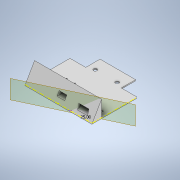
# Autodesk Inventor part: Onixium3
Saved by Autodesk Inventor 2021 (Build 250183000, 183)
## iProperties
Created: 2021-11-17
Part Number: Onixium3
Material: Genérico
Document SubType Name: Chapa
Designer: Juan Camilo
Density: 1 g/cm^3
Sheet Metal Rule: Por defecto_mm
Appearance: Valor por defecto
Author: Juan Camilo
Autodesk Inventor part; units mm, degrees
ref_plane "YZ Plane" through (0, 0, 0) normal (1, 0, 0) x (0, 1, 0)
ref_plane "XZ Plane" through (0, 0, 0) normal (0, 1, 0) x (-1, 0, 0)
ref_plane "XY Plane" through (0, 0, 0) normal (0, 0, 1) x (1, 0, 0)
sketch "Boceto1" plane through (0, 0, 0) normal (0, 1, 0) x (-1, 0, 0)
  line L0 (26, -66) -> (49, -66)
  line L1 (0, -87) -> (0, 0) construction
  line L2 (49, 0) -> (49, -87)
  line L3 (-49, 0) -> (49, 0)
  line L4 (-49, -87) -> (-49, 0)
  line L5 (49, -87) -> (-49, -87)
  line L6 (26, -87) -> (26, -66)
  circle A0 centre (-41.5, -7.5) radius 1.75
  line L7 (49, -12) -> (-49, -12) construction
  circle A1 centre (41.5, -7.5) radius 1.75
  line L8 (-26, -66) -> (-49, -66)
  line L9 (-26, -87) -> (-26, -66)
  line L10 (44.5, -24.05) -> (28.5, -24.05)
  line L11 (28.5, -24.05) -> (28.5, -13.05)
  line L12 (28.5, -13.05) -> (44.5, -13.05)
  line L13 (44.5, -13.05) -> (44.5, -24.05)
  line L14 (42.5, -23.55) -> (31.5, -23.55)
  line L15 (31.5, -14.85) -> (42.5, -14.85)
  line L16 (42.5, -14.85) -> (42.5, -23.55)
  circle A2 centre (30.2, -19.25) radius 1.05
  line L17 (31.5, -14.85) -> (31.5, -23.55)
  line L18 (-42.5, -23.55) -> (-31.5, -23.55)
  line L19 (-42.5, -14.85) -> (-42.5, -23.55)
  line L20 (-31.5, -14.85) -> (-42.5, -14.85)
  line L21 (-31.5, -14.85) -> (-31.5, -23.55)
  circle A3 centre (-30.2, -19.25) radius 1.05
  circle A4 centre (13, -21.5) radius 2.5
  circle A5 centre (-13, -21.5) radius 2.5
  circle A6 centre (16, -70) radius 2.5
  circle A7 centre (-16, -70) radius 2.5
  dimension "d0" = 3.5
  dimension "d1" = 0
  dimension "d2" = 87
  dimension "d3" = 21
  dimension "d4" = 12
  dimension "d5" = 23
  dimension "d6" = 98
  dimension "d7" = 7.5
  dimension "d8" = 7.5
  dimension "d9" = 79.5
  dimension "d10" = 2.1
  dimension "d11" = 9
  dimension "d12" = 11
  dimension "d13" = 16
  dimension "d14" = 1
  dimension "d15" = 3.6
  dimension "d16" = 2.1
  dimension "d17" = 1.3
  dimension "d18" = 5
  dimension "d19" = 36
  dimension "d20" = 9.5
  dimension "d21" = 5
  dimension "d22" = 17
  dimension "d23" = 10
  dimension "d24" = 8.7
  dimension "d25" = 4.3
  dimension "d26" = 4
  dimension "d27" = 11
  dimension "d28" = 54
  dimension "d29" = 2.85
  constraints: 44 end point, 10 symmetric about line, 8 centre point, 5 parallel, 5 point on line, 4 horizontal, 4 perpendicular, 3 midpoint, 1 equal radius, 1 vertical, 3 other
  measures "d0" diameter of A0
  measures "d1" distance of point (0, 0) L1.end
  measures "d2" distance of L2.start L2.end
  measures "d3" distance of L6.start L0.start
  measures "d4" distance between parallel lines of L3 L7
  measures "d5" distance of L0.start L0.end
  measures "d6" distance of L4.end L2.start
  measures "d7" distance from line of L2 A1.centre
  measures "d8" distance from line of L3 A1.centre
  measures "d10" diameter of L7 L12
  measures "d11" diameter of L2 L13
  measures "d12" distance of L11.start L11.end
  measures "d13" distance of L10.start L11.start
  measures "d14" diameter of L14 L10
  measures "d15" diameter of L15 L12
  measures "d16" diameter of A2
  measures "d17" distance from line of L17 A2.centre
  measures "d18" diameter of A4
  measures "d19" distance from line of L2 A4.centre
  measures "d20" distance from line of L7 A4.centre
  measures "d21" diameter of A6
  measures "d22" distance from line of L5 A6.centre
  measures "d23" distance from line of L6 A6.centre
  measures "d24" distance of L17.start L17.end
  measures "d25" distance from line of L14 A2.centre
  measures "d26" diameter of L16 L13
  measures "d27" distance of L17.start L15.end
  measures "d28" distance between parallel lines of L7 L0
  measures "d29" distance between parallel lines of L7 L15
extrude "Base" add sketch "Boceto1" along normal blind 1.5 contours L6 L5 L9 L8 L4 L3 L2 L0 | L10 L11 L12 L13
sketch "Boceto2" plane through (-49, 0, -66) normal (-1, 0, 0) x (0, 0, 1)
  line L0 (66, 0) -> (0, 0)
  line L1 (66, 0) -> (65.1357, 1.5)
  line L2 (66, 0) -> (67.7312, 0) construction
  line L3 (65.1357, 1.5) -> (66, 1.5)
  line L4 (66, 0) -> (66, 1.5)
  line L5 (66, 1.5) -> (66, 0)
  dimension "d32" = 119.95
  constraints: 12 end point, 2 horizontal, 1 equal length, 1 perpendicular
  measures "d32" angle of L2 L1
extrude "Angulo Base" cut sketch "Boceto2" against normal blind 98
sketch "Boceto3" plane through (-49, 0, -66) normal (-1, 0, 0) x (0, 0, 1)
  line L0 (0, 0) -> (66, 0) projected
  line L1 (51.8028, 0) -> (66, 0)
  line L2 (66, 0) -> (51.8028, 24.6399)
  line L3 (51.8028, 24.6399) -> (51.8028, 0)
  line L4 (66, 0) -> (65.1357, 1.5) projected
  dimension "d35" = 0
  constraints: 6 end point, 1 collinear, 1 perpendicular, 1 point on line
  measures "d35" distance between parallel lines of L4 L2
extrude "Extrusión3" add sketch "Boceto3" against normal blind 98
sketch "Boceto4" plane through (-49, 1.5, -14.1972) normal (0, 0, -1) x (-1, 0, 0)
  line L0 (-55.5, 19.6399) -> (-42.5, 19.6399)
  line L1 (-42.5, 19.6399) -> (-42.5, 0.9399)
  line L2 (-42.5, 0.9399) -> (-55.5, 0.9399)
  line L3 (-55.5, 0.9399) -> (-55.5, 19.6399)
  line L4 (-54.6, 10.4399) -> (-43.4, 10.4399)
  line L5 (-43.4, 10.4399) -> (-43.4, 4.8399)
  line L6 (-43.4, 4.8399) -> (-54.6, 4.8399)
  line L7 (-54.6, 4.8399) -> (-54.6, 10.4399)
  line L8 (0, 23.1399) -> (0, 0) projected
  line L9 (-98, 0) -> (-98, 23.1399) projected
  line L10 (0, 23.1399) -> (-98, 23.1399) projected
  line L11 (0, 0) -> (-98, 0) projected
  point P0 (-49, -1.5)
  dimension "d38" = 13
  dimension "d39" = 0.9
  dimension "d40" = 0.9
  dimension "d41" = 3.9
  dimension "d42" = 5.6
  dimension "d43" = 18.7
  dimension "d44" = 42.5
  dimension "d45" = 42.5
  dimension "d46" = 3.5
  dimension "d93" = 0.9399
  constraints: 16 end point, 4 parallel, 2 horizontal, 2 perpendicular
  measures "d38" distance between parallel lines of L1 L3
  measures "d39" distance between parallel lines of L3 L7
  measures "d40" distance between parallel lines of L1 L5
  measures "d41" distance between parallel lines of L2 L6
  measures "d42" distance between parallel lines of L6 L4
  measures "d43" distance between parallel lines of L2 L0
  measures "d44" distance between parallel lines of L8 L1
  measures "d45" distance between parallel lines of L9 L3
  measures "d46" distance between parallel lines of L0 L10
  measures "d93" distance between parallel lines of L11 L2
extrude "Extrusión4" cut sketch "Boceto4" against normal mid plane 76.25 contours L4 L5 L6 L7
sketch "Boceto5" plane through (-49, 1.5, -14.1972) normal (0, 0, -1) x (-1, 0, 0)
  line L0 (-54.6, 19.64) -> (-43.4, 19.64)
  line L1 (-43.4, 19.64) -> (-43.4, 4.84)
  line L2 (-43.4, 4.84) -> (-54.6, 4.84)
  line L3 (-54.6, 4.84) -> (-54.6, 19.64)
  line L4 (-54.6, 4.8399) -> (-54.6, 10.4399) projected
  line L5 (-43.4, 10.4399) -> (-43.4, 4.8399) projected
  line L6 (-43.4, 4.8399) -> (-54.6, 4.8399) projected
  line L7 (-75, 0) -> (-23, 0) projected
  line L8 (0, 23.1399) -> (-98, 23.1399) projected
  point P0 (-49, -1.5)
  dimension "d49" = 11.2
  dimension "d50" = 14.8
  dimension "d76" = 4.84
  constraints: 8 end point, 2 parallel, 1 horizontal, 1 perpendicular
  measures "d49" distance between parallel lines of L1 L3
  measures "d50" distance between parallel lines of L2 L0
  measures "d76" distance between parallel lines of L7 L2
extrude "Extrusión5" cut sketch "Boceto5" against normal mid plane 1.5
sketch "Boceto6" plane through (0, 1.5, 0) normal (0, 1, 0) x (1, 0, 0)
  line L0 (6.5, 13.7984) -> (-6.5, 13.7984)
  line L1 (-6.5, 13.7984) -> (-6.5, 13.8318)
  line L2 (-6.5, 13.8318) -> (6.5, 13.8318)
  line L3 (6.5, 13.8318) -> (6.5, 13.7984)
  line L4 (-6.5, 13.8318) -> (6.5, 13.8318)
  line L5 (6.5, 13.8318) -> (6.5, 18.6972)
  line L6 (6.5, 18.6972) -> (-6.5, 18.6972)
  line L7 (-6.5, 18.6972) -> (-6.5, 13.8318)
  line L8 (-49, 14.1972) -> (49, 14.1972) projected
  point P0 (0, 0)
  point P1 (-6.5, 14.1972)
  point P2 (6.5, 14.1972)
  dimension "d53" = 13
  dimension "d54" = 4.5
  constraints: 16 end point, 4 parallel, 2 horizontal, 2 perpendicular, 1 point on line
  measures "d53" distance between parallel lines of L7 L5
  measures "d54" distance between parallel lines of L8 L6
extrude "Extrusión6" add sketch "Boceto6" along normal blind 20 contours L8 L7 L6 L5
sketch "Boceto7" plane through (6.5, 1.5, -18.6972) normal (0, 0, -1) x (-1, 0, 0)
  line L0 (0.9, 10.916) -> (12.1, 10.916)
  line L1 (12.1, 10.916) -> (12.1, 4.84)
  line L2 (12.1, 4.84) -> (0.9, 4.84)
  line L3 (0.9, 4.84) -> (0.9, 10.916)
  line L4 (13, 0) -> (0, 0) projected
  line L5 (0, 0) -> (0, 20) projected
  line L6 (0.9, 20) -> (12.1, 20)
  line L7 (12.1, 20) -> (12.1, 15.894)
  line L8 (12.1, 15.894) -> (0.9, 15.894)
  line L9 (0.9, 15.894) -> (0.9, 20)
  line L10 (0, 20) -> (13, 20) projected
  point P0 (6.5, -1.5)
  dimension "d57" = 4.84
  dimension "d58" = 6.076
  dimension "d59" = 11.2
  dimension "d60" = 0.9
  dimension "d61" = 4.978
  dimension "d62" = 11.2
  dimension "d63" = 0.9
  dimension "d64" = 0
  constraints: 16 end point, 4 parallel, 2 horizontal, 2 perpendicular
  measures "d57" distance between parallel lines of L4 L2
  measures "d58" distance between parallel lines of L2 L0
  measures "d59" distance between parallel lines of L1 L3
  measures "d60" distance between parallel lines of L5 L3
  measures "d61" distance between parallel lines of L8 L0
  measures "d62" distance between parallel lines of L7 L9
  measures "d63" distance between parallel lines of L5 L9
  measures "d64" distance between parallel lines of L10 L6
extrude "Extrusión7" cut sketch "Boceto7" against normal blind 5.25
sketch "Boceto8" plane through (-5.6, 17.394, -18.6972) normal (0, 1, 0) x (1, 0, 0)
  line L0 (0, 0) -> (0, -4.5) projected
  line L1 (0, -4.5) -> (11.2, -4.5)
  line L2 (11.2, -4.5) -> (11.2, -0.7)
  line L3 (11.2, -0.7) -> (0, -0.7)
  line L4 (0, -0.7) -> (0, -4.5)
  point P0 (5.6, -18.6972)
  point P1 (0, -0.7)
  dimension "d67" = 3.8
  dimension "d68" = 11.2
  constraints: 8 end point, 2 parallel, 1 horizontal, 1 perpendicular
  measures "d67" distance between parallel lines of L3 L1
  measures "d68" distance between parallel lines of L0 L2
extrude "Extrusión8" cut sketch "Boceto8" against normal blind 10.054
sketch "Boceto9" plane through (-5.6, 6.34, -18.6972) normal (0, 1, 0) x (1, 0, 0)
  line L0 (11.2, 0) -> (11.2, -0.7) projected
  line L1 (0, 0) -> (0, -4.5) projected
  line L2 (11.2, -0.7) -> (0, -0.7)
  line L3 (0, -0.7) -> (0, -1.7)
  line L4 (0, -1.7) -> (11.2, -1.7)
  line L5 (11.2, -1.7) -> (11.2, -0.7)
  point P0 (5.6, -18.6972)
  dimension "d77" = 1
  constraints: 8 end point, 2 parallel, 1 horizontal, 1 perpendicular, 1 point on line
  measures "d77" distance between parallel lines of L4 L2
extrude "Extrusión9" cut sketch "Boceto9" against normal blind 3.9
sketch "Boceto12" plane through (0, 1.5, 0) normal (0, 1, 0) x (1, 0, 0)
  line L0 (-49, 0) -> (49, 0) projected
  line L1 (16.0988, 0) -> (49, 15.3421)
  line L2 (49, 0) -> (49, 66) projected
  point P0 (0, 0)
  dimension "d82" = 25
  constraints: 2 end point, 2 point on line
  measures "d82" angle of L0 L1
ref_plane "Plano de trabajo1" through (16.0988, 1.5, 0) normal (-0.4226183, 0, -0.9063078) x (0.9063078, 0, -0.4226183)
sketch "Boceto13" plane through (16.0988, 1.5, 0) normal (-0.4226183, 0, -0.9063078) x (0.9063078, 0, -0.4226183)
  line L0 (20.8186, -18.14) -> (9.6186, -18.14)
  line L1 (9.6186, -18.14) -> (9.6186, 0.56)
  line L2 (9.6186, 0.56) -> (20.8186, 0.56)
  line L3 (20.8186, 0.56) -> (20.8186, -18.14)
  line L4 (22.8276, -9.416) -> (9.6186, -9.416)
  line L5 (9.6186, -9.416) -> (9.6186, -3.34)
  line L6 (9.6186, -3.34) -> (22.8276, -3.34)
  line L7 (22.8276, -3.34) -> (22.8276, -9.416)
  line L8 (35.8186, 0) -> (35.8186, -23.1399) projected
  line L9 (-58.9996, 1.5) -> (29.8186, 1.5) projected
  point P0 (-14.5905, 1.5)
  point P1 (9.6186, -9.416)
  dimension "d84" = 18.7
  dimension "d85" = 11.2
  dimension "d86" = 6.076
  dimension "d87" = 0
  dimension "d88" = 3.9
  dimension "d91" = 15
  dimension "d92" = 0.94
  constraints: 16 end point, 4 parallel, 2 horizontal, 2 perpendicular
  measures "d84" distance between parallel lines of L2 L0
  measures "d85" distance between parallel lines of L1 L3
  measures "d86" distance between parallel lines of L6 L4
  measures "d87" distance between parallel lines of L1 L5
  measures "d88" distance between parallel lines of L2 L6
  measures "d91" distance between parallel lines of L8 L3
  measures "d92" distance between parallel lines of L9 L2
extrude "Extrusión10" cut sketch "Boceto13" against normal mid plane 45.15 contours L4 L1 L6 L3 | L3 L6 L7 L4
equation "\"Radio_pliegue\" = Grosor"
equation "\"Anchura_desahogo_plegado\" = Grosor"
equation "\"Profundidad_desahogo_plegado\" = 0.5 * Grosor"
equation "\"Tamaño_destalonado\" = 4 * Grosor"
equation "\"Remanente_mínimo\" = 2 * Grosor"
equation "\"Radiodetransición\" = Radio_pliegue"
equation "\"Tamaño_de_radio_de_Jacobi\" = Radio_pliegue"
equation "\"TamañoSeparación\" = Grosor"
equation "\"Grosor\" = 0.5"
